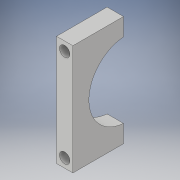
# Autodesk Inventor part: SujetadorColaVTOLv2
Saved by Autodesk Inventor 2019 (Build 230136000, 136)
## iProperties
Created: 2019-03-22
Part Number: SujetadorColaVTOLv2
Material: Generic
Document SubType Name: Modeling
Designer: Kenny
Density: 1 g/cm^3
Appearance: Default
Author: Kenny
Autodesk Inventor part; units mm, degrees
ref_plane "YZ Plane" through (0, 0, 0) normal (1, 0, 0) x (0, 1, 0)
ref_plane "XZ Plane" through (0, 0, 0) normal (0, 1, 0) x (-1, 0, 0)
ref_plane "XY Plane" through (0, 0, 0) normal (0, 0, 1) x (1, 0, 0)
sketch "Sketch1" plane through (0, 0, 0) normal (0, 0, 1) x (1, 0, 0)
  line L0 (0, 0) -> (5.5, 0)
  line L1 (5.5, 0) -> (5.5, 37)
  line L2 (5.5, 37) -> (0, 37)
  line L3 (0, 37) -> (0, 0)
  line L4 (0, 0) -> (5.5, 0)
  line L5 (5.5, 0) -> (5.5, 37)
  line L6 (5.5, 37) -> (0, 37)
  line L7 (0, 37) -> (0, 0)
  line L8 (0, 0) -> (5.5, 0)
  line L9 (5.5, 0) -> (5.5, 37)
  line L10 (5.5, 37) -> (0, 37)
  line L11 (0, 37) -> (0, 0)
  line L12 (0, 0) -> (5.5, 0)
  line L13 (5.5, 0) -> (5.5, 37)
  line L14 (5.5, 37) -> (0, 37)
  line L15 (0, 37) -> (0, 0)
  point P0 (2.75, 34)
  point P1 (2.75, 3)
  point P2 (2.75, 34)
  point P3 (2.75, 3)
  point P4 (2.75, 34)
  point P5 (2.75, 3)
  point P6 (2.75, 34)
  point P7 (2.75, 3)
  dimension "d0" = 5.5
  dimension "d1" = 37
  dimension "d2" = 3
  dimension "d3" = 2.75
  dimension "d4" = 3
  dimension "d5" = 5.5
  dimension "d6" = 37
  dimension "d7" = 3
  dimension "d8" = 2.75
  dimension "d9" = 3
  dimension "d10" = 5.5
  dimension "d11" = 37
  dimension "d12" = 3
  dimension "d13" = 2.75
  dimension "d14" = 3
  dimension "d15" = 5.5
  dimension "d16" = 37
  dimension "d17" = 3
  dimension "d18" = 2.75
  dimension "d19" = 3
  constraints: 32 end point, 8 parallel, 4 horizontal, 4 perpendicular, 4 vertical alignment
  measures "d0" distance of L2.end L1.end
  measures "d1" distance of L1.end L0.end
  measures "d2" distance from line of L2 point (2.75, 34)
  measures "d3" distance from line of L1 point (2.75, 34)
  measures "d4" distance from line of L0 point (2.75, 3)
  measures "d5" distance of L6.end L5.end
  measures "d6" distance of L5.end L4.end
  measures "d7" distance from line of L6 point (2.75, 34)
  measures "d8" distance from line of L5 point (2.75, 34)
  measures "d9" distance from line of L4 point (2.75, 3)
  measures "d10" distance of L10.end L9.end
  measures "d11" distance of L9.end L8.end
  measures "d12" distance from line of L10 point (2.75, 34)
  measures "d13" distance from line of L9 point (2.75, 34)
  measures "d14" distance from line of L8 point (2.75, 3)
  measures "d15" distance of L14.end L13.end
  measures "d16" distance of L13.end L12.end
  measures "d17" distance from line of L14 point (2.75, 34)
  measures "d18" distance from line of L13 point (2.75, 34)
  measures "d19" distance from line of L12 point (2.75, 3)
extrude "Extrusion1" add sketch "Sketch1" along normal blind 17
sketch "Sketch2" plane through (0, 0, 0) normal (0, 0, 1) x (1, 0, 0)
  line L0 (0, 0) -> (5.5, 0)
  line L1 (5.5, 0) -> (5.5, 37)
  line L2 (5.5, 37) -> (0, 37)
  line L3 (0, 37) -> (0, 0)
  line L4 (0, 0) -> (5.5, 0)
  line L5 (5.5, 0) -> (5.5, 37)
  line L6 (5.5, 37) -> (0, 37)
  line L7 (0, 37) -> (0, 0)
  line L8 (0, 0) -> (5.5, 0)
  line L9 (5.5, 0) -> (5.5, 37)
  line L10 (5.5, 37) -> (0, 37)
  line L11 (0, 37) -> (0, 0)
  line L12 (0, 0) -> (5.5, 0)
  line L13 (5.5, 0) -> (5.5, 37)
  line L14 (5.5, 37) -> (0, 37)
  line L15 (0, 37) -> (0, 0)
  point P0 (2.75, 34)
  point P1 (2.75, 3)
  point P2 (2.75, 34)
  point P3 (2.75, 3)
  point P4 (2.75, 34)
  point P5 (2.75, 3)
  point P6 (2.75, 34)
  point P7 (2.75, 3)
  dimension "d20" = 5.5
  dimension "d21" = 37
  dimension "d22" = 3
  dimension "d23" = 2.75
  dimension "d24" = 3
  dimension "d25" = 5.5
  dimension "d26" = 37
  dimension "d27" = 3
  dimension "d28" = 2.75
  dimension "d29" = 3
  dimension "d30" = 5.5
  dimension "d31" = 37
  dimension "d32" = 3
  dimension "d33" = 2.75
  dimension "d34" = 3
  dimension "d35" = 5.5
  dimension "d36" = 37
  dimension "d37" = 3
  dimension "d38" = 2.75
  dimension "d39" = 3
  constraints: 32 end point, 8 parallel, 4 horizontal, 4 perpendicular, 4 vertical alignment
  measures "d20" distance of L2.end L1.end
  measures "d21" distance of L1.end L0.end
  measures "d22" distance from line of L2 point (2.75, 34)
  measures "d23" distance from line of L1 point (2.75, 34)
  measures "d24" distance from line of L0 point (2.75, 3)
  measures "d25" distance of L6.end L5.end
  measures "d26" distance of L5.end L4.end
  measures "d27" distance from line of L6 point (2.75, 34)
  measures "d28" distance from line of L5 point (2.75, 34)
  measures "d29" distance from line of L4 point (2.75, 3)
  measures "d30" distance of L10.end L9.end
  measures "d31" distance of L9.end L8.end
  measures "d32" distance from line of L10 point (2.75, 34)
  measures "d33" distance from line of L9 point (2.75, 34)
  measures "d34" distance from line of L8 point (2.75, 3)
  measures "d35" distance of L14.end L13.end
  measures "d36" distance of L13.end L12.end
  measures "d37" distance from line of L14 point (2.75, 34)
  measures "d38" distance from line of L13 point (2.75, 34)
  measures "d39" distance from line of L12 point (2.75, 3)
hole "Hole1" at (2.75, 34, 0) at (2.75, 3, 0) direction (0, 0, 1) diameter 3.5 end through all
sketch "Sketch3" plane through (5.5, 0, 0) normal (1, 0, 0) x (0, 0, -1)
  line L0 (0, 0) -> (-17, 0) projected
  line L1 (-17, 0) -> (1, 0)
  line L2 (1, 0) -> (1, 37)
  line L3 (1, 37) -> (-17, 37)
  line L4 (-17, 37) -> (-17, 0)
  arc A0 (1, 31.125) -> (1, 5.875) centre (1, 18.5) ccw
  dimension "d49" = 18
  dimension "d50" = 25.25
  constraints: 8 end point, 2 parallel, 2 point on circle, 2 point on line, 1 centre point, 1 horizontal, 1 midpoint, 1 perpendicular
  measures "d49" distance of L3.end L2.end
  measures "d50" diameter of A0
extrude "Extrusion2" cut sketch "Sketch3" against normal blind 5.5 contours A0 L2
body "Solid1"
